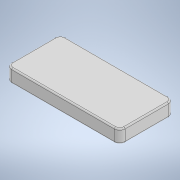
# Autodesk Inventor part: mattress
Saved by Autodesk Inventor 2022 (Build 260153000, 153)
## iProperties
Created: 2022-04-19
Part Number: mattress
Material: Generic
Document SubType Name: Modeling
Designer: compsci
Density: 1 g/cm^3
Appearance: Default
Author: compsci
Autodesk Inventor part; units mm, degrees
ref_plane "YZ Plane" through (0, 0, 0) normal (1, 0, 0) x (0, 1, 0)
ref_plane "XZ Plane" through (0, 0, 0) normal (0, 1, 0) x (-1, 0, 0)
ref_plane "XY Plane" through (0, 0, 0) normal (0, 0, 1) x (1, 0, 0)
sketch "Sketch1" plane through (0, 0, 0) normal (0, 1, 0) x (-1, 0, 0)
  line L0 (1066.8, 508) -> (-1066.8, 508)
  line L1 (-1066.8, 508) -> (-1066.8, -508)
  line L2 (-1066.8, -508) -> (1066.8, -508)
  line L3 (1066.8, -508) -> (1066.8, 508)
  line L4 (1066.8, 508) -> (-1066.8, -508) construction
  line L5 (-1066.8, 508) -> (1066.8, -508) construction
  point P0 (0, 0)
  dimension "d0" = 1016
  dimension "d1" = 2133.6
  constraints: 12 end point, 2 midpoint, 2 parallel, 1 horizontal, 1 perpendicular
  measures "d0" distance of L0.end L1.end
  measures "d1" distance of L1.end L2.end
extrude "Extrusion1" add sketch "Sketch1" along normal blind 254
fillet "Fillet1" radius 101.6 4 edges at (1066.8, 127, 508) (1066.8, 127, -508) (-1066.8, 127, 508) (-1066.8, 127, -508)
fillet "Fillet2" radius 25.4 16 edges at (-1037.042, 254, -478.242) (-1066.8, 254, 0) (-1037.042, 254, 478.242) (0, 254, 508) (1037.042, 254, 478.242) (1066.8, 254, 0) (1037.042, 254, -478.242) (0, 254, -508) (-1037.042, 0, -478.242) (-1066.8, 0, 0) (-1037.042, 0, 478.242) (0, 0, 508) (1037.042, 0, 478.242) (1066.8, 0, 0) (1037.042, 0, -478.242) (0, 0, -508)
body "Solid1"
